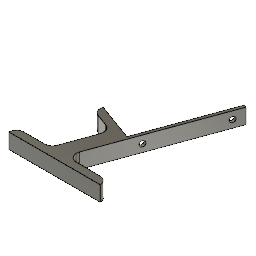
DisplayEnclosure_VerticalStand_v1 (Autodesk Fusion 360 design; units mm, degrees)
Autodesk Fusion 360 part; units mm, degrees
sketch "Sketch1" plane through (0, 0, 0) normal (0, 0, 1) x (1, 0, 0)
  line L0 (0, 0) -> (60, 0)
  line L1 (60, 0) -> (60, 5)
  line L2 (60, 5) -> (0, 5)
  line L3 (0, 5) -> (0, 0)
  line L4 (30, 5) -> (30, 45) construction
  line L5 (30, 5) -> (32.128, 5) construction
  line L6 (32.128, 5) -> (63.7225, 91.8051)
  line L7 (32.128, 5) -> (188.367, 5) construction
  line L8 (30, 5) -> (61.8434, 92.489) construction
  line L9 (30, 5) -> (186.3489, 5) construction
  line L10 (41.3222, 36.1075) -> (16.8902, 45)
  line L11 (30, 45) -> (0, 45) construction
  line L12 (16.8902, 45) -> (15.1801, 40.3015)
  line L13 (32.128, 5) -> (22.128, 5) construction
  line L14 (15.1801, 40.3015) -> (39.6121, 31.409) construction
  line L15 (22.128, 5) -> (32.6609, 33.939)
  line L16 (22.128, 5) -> (52.84, 5) construction
  line L17 (41.3222, 36.1075) -> (61.8434, 92.489)
  line L18 (30, 5) -> (32.128, 5) construction
  line L19 (61.8434, 92.489) -> (63.7225, 91.8051)
  line L20 (15.1801, 40.3015) -> (32.6609, 33.939)
  dimension "d1" = 60
  dimension "d2" = 5
  dimension "d3" = 40
  dimension "d4" = 2.128
  dimension "d5" = 70
  dimension "d6" = 70
  dimension "d7" = 26
  dimension "d8" = 5
  dimension "d9" = 10
  dimension "d10" = 70
  dimension "d11" = 60
  constraint horizontal L0
  constraint vertical L1
  constraint horizontal L2
  constraint vertical L3
  constraint coincident L0.start L3.end
  constraint midpoint L2 L4.start
  constraint perpendicular L2 L4
  constraint perpendicular L4 L5
  constraint horizontal L7
  constraint horizontal L9
  constraint coincident L8 L10.start
  constraint perpendicular L8 L10
  constraint perpendicular L4 L11
  constraint coincident L10.end L11
  constraint perpendicular L10 L12
  constraint parallel L2 L13
  constraint coincident L8 L14.end
  constraint perpendicular L8 L14
  constraint horizontal L16
  constraint coincident L14 L15.end
  constraint perpendicular L10 L17
  constraint coincident L8.end L17.end
  constraint coincident L6 L19.end
  constraint perpendicular L6 L19
  constraint coincident L6.end L19.end
  measures "d1" distance of L0.start L0.end
  measures "d2" distance of L0.start L2.end
  measures "d3" distance of L4.start L4.end
  measures "d4" distance of L4.start L5.end
  measures "d5" angle of L6 L7
  measures "d6" angle of L8 L9
  measures "d7" distance of L10.start L10.end
  measures "d8" distance of L10.end L12.end
  measures "d9" distance of L5.end L13.end
  measures "d10" angle of L15 L16
  measures "d11" distance of L10.start L8.end
extrude "Extrude1" add sketch "Sketch1" along normal blind 10
fillet "Fillet1" radius 5 1 edges at (22.128, 5, 5)
fillet "Fillet2" radius 5 1 edges at (32.128, 5, 5)
fillet "Fillet3" radius 5 1 edges at (32.6609, 33.939, 5)
fillet "Fillet4" radius 5 1 edges at (0, 5, 5)
fillet "Fillet5" radius 5 1 edges at (60, 5, 5)
fillet "Fillet6" radius 5 1 edges at (15.1801, 40.3015, 5)
sketch "Sketch2" plane through (24.8837, -9.0569, 0) normal (-0.939693, 0.34202, 0) x (-0.34202, -0.939693, 0)
  line L0 (-108.063, 0) -> (-48.063, 0)
  line L1 (-48.063, 0) -> (-48.063, 10)
  line L2 (-48.063, 10) -> (-108.063, 10)
  line L3 (-108.063, 10) -> (-108.063, 0)
  line L4 (-108.063, 5) -> (-101.063, 5) construction
  line L5 (-101.063, 5) -> (-55.063, 5) construction
  circle A0 centre (-55.063, 5) radius 1.75
  circle A1 centre (-101.063, 5) radius 1.75
  dimension "d26" = 7
  dimension "d27" = 46
  dimension "d28" = 3.5
  dimension "d29" = 3.5
  constraint midpoint L3 L4.start
  constraint perpendicular L3 L4
  constraint parallel L4 L5
  constraint coincident L5.end A0.centre
  constraint coincident L4.end L5.start
  measures "d26" distance of L4.start L4.end
  measures "d27" distance of L4.end L5.end
  measures "d28" diameter of A0
  measures "d29" diameter of A1
extrude "Extrude2" cut sketch "Sketch2" against normal blind 2 contours A0 | A1
